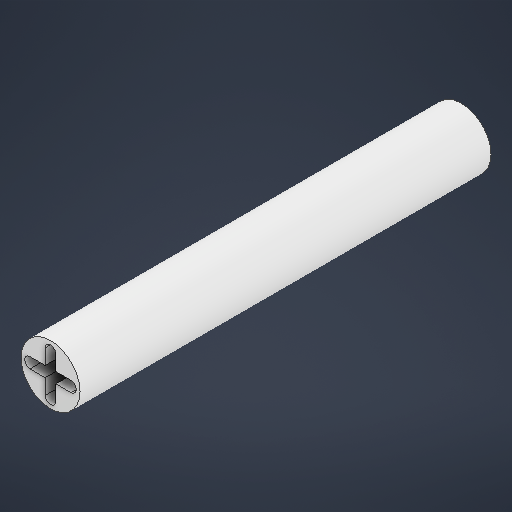
# Autodesk Inventor part: Tussen stuk V1.1
Saved by Autodesk Inventor 2026.2 (Build 302298000, 298)
## iProperties
Created: 2026-05-03
Part Number: Tussen stuk V1.1
Material: ABS Plastic
Document SubType Name: Modeling
Designer: Gameb
Density: 1.06 g/cm^3
Appearance: Smooth - White
Author: Gameb
Autodesk Inventor part; units mm, degrees
ref_plane "YZ Plane" through (0, 0, 0) normal (1, 0, 0) x (0, 1, 0)
ref_plane "XZ Plane" through (0, 0, 0) normal (0, 1, 0) x (-1, 0, 0)
ref_plane "XY Plane" through (0, 0, 0) normal (0, 0, 1) x (1, 0, 0)
sketch "Sketch1" plane through (0, 0, 0) normal (0, 0, 1) x (1, 0, 0)
  line L0 (-8, -2) -> (-2, -2)
  line L1 (-2, -2) -> (-8, -2)
  line L2 (-2, -2) -> (-2, -7.923)
  line L3 (2, -8) -> (2, -2.0038)
  line L4 (2, -2.0038) -> (2, -8)
  arc A0 (8, -2.0038) -> (10.0019, 0) centre (8, -0.0019) ccw
  line L5 (2, -2.0038) -> (8, -2.0038)
  line L6 (2, 2) -> (2, 8)
  line L7 (8, 2) -> (2, 2)
  line L8 (2, 2) -> (8, 2)
  line L9 (2, 2) -> (2, 8)
  line L10 (-2, 8) -> (-2, 2)
  line L11 (-2, 2) -> (-2, 8)
  arc A1 (-8, 2) -> (-10, 0) centre (-8, 0) ccw
  line L12 (-2, 2) -> (-8, 2)
  arc A2 (-8, 2) -> (-8, -2) centre (-8, 0) ccw
  arc A3 (-2, -8) -> (0, -10) centre (0, -8) ccw
  arc A4 (-2, -8) -> (2, -8) centre (0, -8) ccw
  arc A5 (8, -2.0038) -> (8, 2) centre (8, -0.0019) ccw
  arc A6 (2, 8) -> (-2, 8) centre (0, 8) ccw
  circle A7 centre (0, 0) radius 11.5
  line L13 (-2, 2) -> (-2.3536, 2.3536)
  line L14 (-2, 2) -> (-1.5, 2) construction
  line L15 (-2.3536, 2.3536) -> (-8, 2.3536)
  line L16 (-8, 2.3536) -> (-8, 2)
  line L17 (-2, -2) -> (-2.3536, -2.3536)
  line L18 (-2.3536, -2.3536) -> (-8, -2.3536)
  line L19 (-8, -2.3536) -> (-8, -2)
  line L20 (-2.3536, -2.3536) -> (-2.3536, -8)
  line L21 (-2.3536, -8) -> (-2, -8)
  line L22 (2, -2.0038) -> (2.3536, -2.3573)
  line L23 (2.3536, -2.3573) -> (2.3536, -8)
  line L24 (2.3536, -8) -> (2, -8)
  line L25 (-2, -7.923) -> (-2, -8)
  line L26 (2.3536, -2.3573) -> (8, -2.3573)
  line L27 (8, -2.3573) -> (8, -2.0038)
  line L28 (2, 2) -> (2.3536, 2.3536)
  line L29 (2.3536, 2.3536) -> (8, 2.3536)
  line L30 (8, 2.3536) -> (8, 2)
  line L31 (2.3536, 2.3536) -> (2.3536, 8)
  line L32 (2.3536, 8) -> (2, 8)
  line L33 (-2.3536, 2.3536) -> (-2.3536, 8)
  line L34 (-2.3536, 8) -> (-2, 8)
  arc A8 (2.3536, 8) -> (-2.3536, 8) centre (0, 8) ccw
  arc A9 (8, -2.3573) -> (8, 2.3536) centre (8, -0.0019) ccw
  arc A10 (-2.3536, -8) -> (2.3536, -8) centre (0, -8) ccw
  arc A11 (-8, 2.3536) -> (-8, -2.3536) centre (-8, 0) ccw
  line L35 (-2, 2) -> (-2.0707, 2.0707)
  line L36 (-2.0707, 2.0707) -> (-8, 2.0707)
  line L37 (-2.0707, 2.0707) -> (-2.0707, 8)
  line L38 (-2, -2) -> (-2.0707, -2.0707)
  line L39 (-2.0707, -2.0707) -> (-8, -2.0707)
  line L40 (-2.0707, -2.0707) -> (-2.0354, -8)
  line L41 (2, -2.0038) -> (2.0707, -2.0745)
  line L42 (2.0707, -2.0745) -> (2.0707, -8)
  line L43 (2.0707, -2.0745) -> (8, -2.0745)
  line L44 (2, 2) -> (2.0707, 2.0707)
  line L45 (2.0707, 2.0707) -> (8, 2.0707)
  line L46 (2.0707, 2.0707) -> (2.0707, 8)
  arc A12 (2.0707, 8) -> (-2.0707, 8) centre (0, 8) ccw
  arc A13 (-8, 2.0707) -> (-8, -2.0707) centre (-8, 0) ccw
  arc A14 (-2.0354, -8) -> (2.0707, -8) centre (0.0177, -8) ccw
  arc A15 (8, -2.0745) -> (8, 2.0707) centre (8, -0.0019) ccw
  dimension "d1" = 23
  dimension "d2" = 0.5
  dimension "d3" = 135
  dimension "d4" = 0.5
  dimension "d6" = 5.6464
  dimension "d7" = 5.6464
  dimension "d8" = 0.5
  dimension "d9" = 0.5
  dimension "d10" = 0.1
  dimension "d11" = 0.1
  dimension "d13" = 0.1
  dimension "d14" = 0.1
  constraints: 94 end point, 33 point on circle, 22 tangent, 20 perpendicular, 20 point on line, 16 centre point, 6 horizontal, 3 collinear, 1 coincident, 1 equal length, 1 parallel, 1 vertical
  measures "d1" diameter of A7
  measures "d2" distance of L12.start L13.end
  measures "d3" angle of L14 L13
  measures "d4" distance of L0.end L17.end
  measures "d6" distance of L13.end L15.end
  measures "d7" distance of L17.end L18.end
  measures "d8" distance of L3.end L22.end
  measures "d9" distance of L9.start L28.end
  measures "d10" distance of L12.start L35.end
  measures "d11" distance of L0.end L38.end
  measures "d13" distance of L3.end L41.end
  measures "d14" distance of L9.start L44.end
extrude "Extrusion1" add sketch "Sketch1" along normal blind 10 contours L39 L17 L18 L19 | L19 A11 L16 A13 | L40 L21 L20 L17 | L16 L15 L13 L36 | A14 L24 A10 L21 | L13 L33 L34 L37 | L42 L22 L23 L24 | L34 A8 L32 A12 | L43 L27 L26 L22 | L32 L31 L28 L46 | A15 L30 A9 L27 | L28 L29 L30 L45 | A7
extrude "Extrusion2" add sketch "Sketch1" against normal blind 150 contours A2 A1 L12 L10 A6 L6 L7 A5 A0 L5 L3 A4 A3 L25 L2 L0 | L19 A13 L16 A1 A2 | L0 L17 L39 L19 | L2 L25 L21 L40 L17 | L39 L17 L18 L19 | L19 A11 L16 A13 | L40 L21 L20 L17 | L16 L36 L13 L12 | L16 L15 L13 L36 | A3 A4 L24 A14 L21 | A14 L24 A10 L21 | L13 L37 L34 L10 | L13 L33 L34 L37 | L42 L22 L23 L24 | L24 L3 L22 L42 | L34 A12 L32 A6 | L34 A8 L32 A12 | L43 L27 L26 L22 | L22 L5 L27 L43 | L32 L46 L28 L6 | L32 L31 L28 L46 | A15 L30 A9 L27 | L27 A0 A5 L30 A15 | L28 L45 L30 L7 | L28 L29 L30 L45 | A7
sketch "Sketch2" plane through (0, 0, -150) normal (0, 0, -1) x (-1, 0, 0)
  circle A0 centre (0, 0) radius 2.3
  dimension "d19" = 4.6
  constraints: 1 centre point, 1 coincident
  measures "d19" diameter of A0
extrude "Extrusion3" cut sketch "Sketch2" against normal blind 6
body "Solid1"
